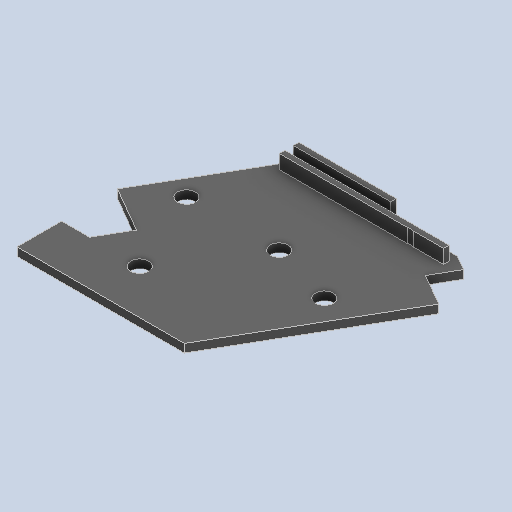
# Autodesk Inventor part: rail_cover_under
Saved by Autodesk Inventor 2024.1 (Build 281209000, 209)
## iProperties
Created: 2025-01-17
Part Number: rail_cover_under
Material: 一般
Document SubType Name: モデリング
Designer: hibik
Density: 1 g/cm^3
Appearance: 既定
Sheet Metal Rule: Default_mm
Author: hibik
Autodesk Inventor part; units mm, degrees
ref_plane "YZ Plane" through (0, 0, 0) normal (1, 0, 0) x (0, 1, 0)
ref_plane "XZ Plane" through (0, 0, 0) normal (0, 1, 0) x (-1, 0, 0)
ref_plane "XY Plane" through (0, 0, 0) normal (0, 0, 1) x (1, 0, 0)
sketch "スケッチ1" plane through (0, 0, 0) normal (0, 1, 0) x (-1, 0, 0)
  line L0 (0, 0) -> (30, 0)
  line L1 (30, 0) -> (30, -135.2775)
  line L2 (30, -135.2775) -> (-78.1025, -135.2775)
  line L3 (-78.1025, -135.2775) -> (0, 0)
  dimension "d0" = 30
  dimension "d1" = 60
  constraints: 8 end point, 2 horizontal, 1 vertical
  measures "d0" distance of L0.start L0.end
  measures "d1" angle of L0 L3
extrude "押し出し1" add sketch "スケッチ1" along normal blind 1.5
sketch "スケッチ2" plane through (0, 1.5, 0) normal (0, 1, 0) x (1, 0, 0)
  line L0 (-25, 8) -> (-25, 1.5) projected
  line L1 (-21.9199, 13.3349) -> (-25, 8) projected
  line L2 (-30, 18) -> (-21.9199, 13.3349) projected
  line L3 (-24.2265, 28) -> (-30, 18) projected
  line L4 (0, 28) -> (-24.2265, 28) projected
  line L5 (0, 36.5) -> (0, 28) projected
  line L6 (5, 36.5) -> (0, 36.5) projected
  line L7 (5, 38) -> (5, 36.5) projected
  line L8 (10.9697, 38) -> (5, 38) projected
  line L9 (13.5677, 36.5) -> (10.9697, 38) projected
  line L10 (11.0677, 32.1699) -> (13.5677, 36.5) projected
  line L11 (16.6969, 28.9199) -> (11.0677, 32.1699) projected
  line L12 (7.3612, 12.75) -> (16.6969, 28.9199) projected
  line L13 (0, 17) -> (7.3612, 12.75) projected
  line L14 (-12, 17) -> (0, 17) projected
  line L15 (-12, 8) -> (-12, 17) projected
  line L16 (-5, 8) -> (-12, 8) projected
  line L17 (-5, 1.5) -> (-5, 8) projected
  line L18 (-25, 1.5) -> (-5, 1.5) projected
  line L19 (78.1025, 135.2775) -> (-30, 135.2775) projected
  line L20 (-30, 135.2775) -> (-30, 0) projected
  line L21 (-30, 0) -> (0, 0) projected
  line L22 (0, 0) -> (78.1025, 135.2775) projected
  line L23 (-24.2265, 28) -> (-18.453, 38)
  line L24 (-18.453, 38) -> (5, 38)
  line L25 (13.5677, 36.5) -> (19.1969, 33.25)
  constraints: 6 end point, 1 collinear, 1 horizontal, 1 perpendicular, 1 point on line
extrude "押し出し2" cut sketch "スケッチ2" against normal through all contours L20 L19 L22 L25 L9 L8 L24 L23 L3
sketch "スケッチ3" plane through (0, 1.5, 0) normal (0, 1, 0) x (1, 0, 0)
  line L0 (-30, 18) -> (-21.9199, 13.3349) projected
  line L1 (-21.9199, 13.3349) -> (-25, 8) projected
  line L2 (-25, 8) -> (-30, 8)
  line L3 (-30, 18) -> (-30, 0) projected
  line L4 (11.0677, 32.1699) -> (13.5677, 36.5) projected
  line L5 (16.6969, 28.9199) -> (11.0677, 32.1699) projected
  line L6 (19.1969, 33.25) -> (10.9697, 38) projected
  line L7 (0, 0) -> (19.1969, 33.25) projected
  constraints: 2 end point, 1 horizontal, 1 point on line
extrude "押し出し3" cut sketch "スケッチ3" against normal through all
sketch "スケッチ4" plane through (0, 0, 0) normal (0, -1, 0) x (1, 0, 0)
  line L0 (-18.453, -39) -> (10.9697, -39) projected
  line L1 (-18.453, -38) -> (-18.453, -39) projected
  line L2 (-18.453, -39) -> (10.9697, -39) projected
  line L3 (10.9697, -39) -> (10.9697, -38) projected
  line L4 (10.9697, -38) -> (-18.453, -38) projected
  line L5 (-18.453, -36.5) -> (10.9697, -36.5) projected
  line L6 (10.9697, -36.5) -> (10.9697, -35.5) projected
  line L7 (10.9697, -35.5) -> (5.5568, -35.5) projected
  line L8 (-18.453, -35.5) -> (-18.453, -36.5) projected
  line L9 (-1, -38) -> (-1, -36.5) projected
  line L10 (-1, -39) -> (-1, -35.5)
  arc A0 (4.4432, -35.5) -> (5.5568, -35.5) centre (5, -34) ccw projected
  line L11 (4.4432, -35.5) -> (-18.453, -35.5) projected
  point P0 (0, 0)
  constraints: 2 end point, 2 point on line, 1 collinear, 1 perpendicular
extrude "押し出し4" add sketch "スケッチ4" against normal blind 4 contours L1 L4 L10 L0 | L8 L11 L10 L5 | L10 L11 A0 L7 L6 L5
sketch "スケッチ5" plane through (0, 0, 0) normal (0, -1, 0) x (1, 0, 0)
  circle A0 centre (-6, -23) radius 1.35 projected
  circle A1 centre (5.5311, -19.5801) radius 1.35 projected
  circle A2 centre (-16, -8) radius 1.35 projected
  circle A3 centre (-22.5359, -22.9282) radius 1.35 projected
  circle A4 centre (-22.5359, -22.9282) radius 1.6
  circle A5 centre (-16, -8) radius 1.6
  circle A6 centre (-6, -23) radius 1.6
  circle A7 centre (5.5311, -19.5801) radius 1.6
  point P0 (0, 0)
  dimension "d13" = 3.2
  constraints: 4 centre point, 4 coincident, 3 equal radius
  measures "d13" diameter of A4
extrude "押し出し5" cut sketch "スケッチ5" against normal through all contours A0 | A1 | A2 | A3 | A4 | A5 | A6 | A7
equation "\"BendRadius\" = Thickness"
equation "\"BendReliefWidth\" = Thickness"
equation "\"BendReliefDepth\" = 0.5 * Thickness"
equation "\"CornerReliefSize\" = 4 * Thickness"
equation "\"MinimumRemnant\" = 2 * Thickness"
equation "\"TransitionRadius\" = BendRadius"
equation "\"JacobiRadiusSize\" = BendRadius"
equation "\"GapSize\" = Thickness"
equation "\"d6\" = Thickness"
equation "\"Thickness\" = 1.5"
